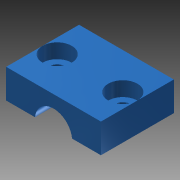
# Autodesk Inventor part: ZAxisRodClampTop
Saved by Autodesk Inventor 2015 SP1 (Build 190203100, 203)
## iProperties
Category: Print
Created: 2014-08-22
Part Number: ZAxisRodClampTop
Material: ABS Plastic
Document SubType Name: Modeling
Designer: t_clevj
Density: 1.06 g/cm^3
Appearance: Cyan
Mass: 3.24999 g
Surface Area: 20.2877 cm^2
Volume: 3.06603 cm^3
Vendor: Jack
Author: Jack
Autodesk Inventor part; units mm, degrees
ref_plane "YZ Plane" through (0, 0, 0) normal (1, 0, 0) x (0, 1, 0)
ref_plane "XZ Plane" through (0, 0, 0) normal (0, 1, 0) x (-1, 0, 0)
ref_plane "XY Plane" through (0, 0, 0) normal (0, 0, 1) x (1, 0, 0)
sketch "Sketch1" plane through (0, 0, 0) normal (0, 1, 0) x (-1, 0, 0)
  circle A0 centre (0, -0.5) radius 5.1
  line L0 (5.0754, 0) -> (13, 0)
  line L1 (13, 0) -> (13, 8)
  line L2 (13, 8) -> (-13, 8)
  line L3 (-13, 8) -> (-13, 0)
  line L4 (-13, 0) -> (-5.0754, 0)
  point P0 (0, 0)
  dimension "d0" = 10.2
  dimension "d1" = 0.5
  dimension "d2" = 26
  dimension "d3" = 13
  dimension "d4" = 8
  constraints: 10 end point, 3 perpendicular, 2 point on circle, 2 point on line, 1 centre point, 1 horizontal, 1 horizontal alignment, 1 vertical alignment
  measures "d0" diameter of A0
  measures "d1" distance of point (0, 0) A0.centre
  measures "d2" distance of L1.end L2.end
  measures "d3" distance from line of point (0, 0) L3
  measures "d4" distance between parallel lines of L0 L2
extrude "Extrusion1" add sketch "Sketch1" along normal blind 20 contours A0 L4 L3 L2 L1 L0
sketch "Sketch2" plane through (-5.0754, 0, 0) normal (0, 0, -1) x (-1, 0, 0)
  line L0 (0, 0) -> (7.9246, 0) projected
  line L1 (7.9246, 0) -> (7.9246, 20) projected
  line L2 (-18.0754, 0) -> (-10.1509, 0) projected
  line L3 (-10.1509, 0) -> (-10.1509, 20) projected
  line L4 (-18.0754, 20) -> (-10.1509, 20) projected
  line L5 (-18.0754, 0) -> (-18.0754, 20) projected
  circle A0 centre (-14.0754, 10) radius 2.25
  circle A1 centre (3.9246, 10) radius 2.25
  point P0 (-5.0754, 0)
  dimension "d8" = 4.5
  dimension "d9" = 18
  dimension "d10" = 4
  dimension "d11" = 10
  constraints: 2 centre point, 1 equal radius, 1 horizontal alignment
  measures "d8" diameter of A1
  measures "d9" distance of A0.centre A1.centre
  measures "d10" distance from line of L1 A1.centre
  measures "d11" distance from line of L0 A1.centre
extrude "Extrusion2" cut sketch "Sketch2" against normal up to surface (8 mm away) contours A0 | A1
sketch "Sketch3" plane through (-13, 0, 8) normal (0, 0, 1) x (1, 0, 0)
  circle A0 centre (4, 10) radius 2.25 projected
  circle A1 centre (22, 10) radius 2.25 projected
  circle A2 centre (4, 10) radius 2.25 projected
  circle A3 centre (4, 10) radius 4
  circle A4 centre (22, 10) radius 4
  point P0 (13, 0)
  dimension "d14" = 8
  constraints: 2 centre point, 2 coincident, 1 equal radius
  measures "d14" diameter of A3
extrude "Extrusion3" cut sketch "Sketch3" against normal blind 4
body "Solid1"
